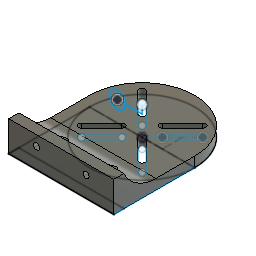
panto (Autodesk Fusion 360 archive; units mm, degrees)
design "support"
Autodesk Fusion 360 part; units mm, degrees
sketch "Esquisse1" plane through (0, 0, 0) normal (0, 1, 0) x (1, 0, 0)
  circle A0 centre (0, 0) radius 26
  line L0 (0, 0) -> (-26, 0) construction
  line L1 (0, 0) -> (26, 0) construction
  line L2 (-26, 0) -> (26, 0)
  line L3 (26, 0) -> (26, -40)
  line L4 (26, -40) -> (-26, -40)
  line L5 (-26, -40) -> (-26, 0)
  line L6 (-26, -40) -> (26, -40)
  line L7 (26, -40) -> (26, -35)
  line L8 (26, -35) -> (-26, -35)
  line L9 (-26, -35) -> (-26, -40)
  line L10 (0, 0) -> (15, 15)
  line L11 (13.9393, 16.0607) -> (3.9393, 6.0607)
  arc A1 (3.9393, 6.0607) -> (6.0607, 3.9393) centre (5, 5) ccw
  line L12 (6.0607, 3.9393) -> (16.0607, 13.9393)
  arc A2 (16.0607, 13.9393) -> (13.9393, 16.0607) centre (15, 15) ccw
  line L13 (15, 15) -> (5, 5) construction
  line L14 (0, 0) -> (10, 0) construction
  line L15 (10, 0) -> (10, 10) construction
  line L16 (-3.9393, 6.0607) -> (-13.9393, 16.0607)
  arc A3 (-6.0607, 3.9393) -> (-3.9393, 6.0607) centre (-5, 5) ccw
  line L17 (-16.0607, 13.9393) -> (-6.0607, 3.9393)
  arc A4 (-13.9393, 16.0607) -> (-16.0607, 13.9393) centre (-15, 15) ccw
  line L18 (-6.0607, -3.9393) -> (-16.0607, -13.9393)
  arc A5 (-3.9393, -6.0607) -> (-6.0607, -3.9393) centre (-5, -5) ccw
  line L19 (-13.9393, -16.0607) -> (-3.9393, -6.0607)
  arc A6 (-16.0607, -13.9393) -> (-13.9393, -16.0607) centre (-15, -15) ccw
  line L20 (3.9393, -6.0607) -> (13.9393, -16.0607)
  arc A7 (6.0607, -3.9393) -> (3.9393, -6.0607) centre (5, -5) ccw
  line L21 (16.0607, -13.9393) -> (6.0607, -3.9393)
  arc A8 (13.9393, -16.0607) -> (16.0607, -13.9393) centre (15, -15) ccw
  dimension "d1" = 52
  dimension "d2" = 40
  dimension "d3" = 5
  dimension "d4" = 3
  dimension "d5" = 10
  dimension "d7" = 360
  constraint coincident A0.centre L0.start
  constraint coincident A0 L0.end
  constraint horizontal L0
  constraint coincident A0 L1.end
  constraint parallel L0 L1
  constraint horizontal L2
  constraint vertical L3
  constraint horizontal L4
  constraint vertical L5
  constraint horizontal L6
  constraint vertical L7
  constraint horizontal L8
  constraint vertical L9
  constraint coincident L3 L7.end
  constraint tangent L11 A1
  constraint tangent A1 L12
  constraint parallel L11 L12
  constraint tangent L12 A2
  constraint tangent L11 A2
  constraint coincident L10 A1.centre
  constraint parallel L10 L13
  constraint coincident L10.end A2.centre
  constraint parallel L1 L14
  constraint midpoint L13 L15.end
  constraint perpendicular L14 L15
  measures "d1" diameter of A0
  measures "d2" distance of L0.end L4.end
  measures "d3" distance of L4.end L8.end
  measures "d4" diameter of A1
  measures "d5" distance of A0.centre L14.end
extrude "Extrusion1" add sketch "Esquisse1" along normal blind 5 contours A0 L2 | A0 L3 L5 L8 | A0 L2
extrude "Extrusion2" add sketch "Esquisse1" along normal blind 15 contours L3 L4 L5 L6 L7 L8 L9
fillet "Congé1" radius 17.5 1 edges at (0, 5, 35)
sketch "Esquisse2" plane through (0, 0, 0) normal (0, 0, 1) x (1, 0, 0)
  line L0 (0, 10) -> (-12.25, 10)
  circle A0 centre (-12.25, 10) radius 1.5
  circle A1 centre (-12.25, 10) radius 4
  line L1 (0, 10) -> (0, 14)
  dimension "d14" = 12.25
  dimension "d15" = 3
  dimension "d16" = 8
  constraint horizontal L0
  constraint coincident L0.end A0.centre
  constraint concentric A0 A1
  constraint perpendicular L0 L1
  measures "d14" distance of L0.start L0.end
  measures "d15" diameter of A0
  measures "d16" diameter of A1
extrude "Extrusion3" cut sketch "Esquisse2" along normal blind 73 contours A0
extrude "Extrusion4" cut sketch "Esquisse2" along normal blind 35
mirror "Symétrie miroir1" about plane through (0, 0, 0) normal (1, 0, 0) of "Extrusion4"
mirror "Symétrie miroir2" about plane through (0, 0, 0) normal (1, 0, 0) of "Extrusion3"
equation "d2 = 66 mm - 26 mm"

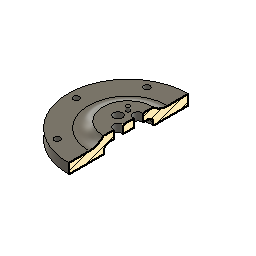
design "liaison"
Autodesk Fusion 360 part; units mm, degrees
sketch "Esquisse1" plane through (0, 0, 0) normal (0, 1, 0) x (1, 0, 0)
  circle A0 centre (5, 0) radius 2.25
  circle A1 centre (12.7279, 12.7279) radius 3
  spline S0 degree 3 poles (12.0292, -14.0552) (11.9758, -14.0271) (11.9242, -13.9959) (11.7208, -13.8551) (11.5886, -13.7213) (11.3733, -13.402) (11.2964, -13.2175) (11.2197, -12.8368) (11.2181, -12.6441) (11.2823, -12.2958) (11.3379, -12.1407) (11.4634, -11.9156) (11.5166, -11.8383) (11.5925, -11.7474) (11.6089, -11.7288) (11.6353, -11.7002) (11.645, -11.6899) (11.6633, -11.6711) (11.6718, -11.6626) (11.6907, -11.6442) (11.7011, -11.6344) (11.7308, -11.607) (11.7504, -11.5899) (11.8478, -11.5091) (11.9313, -11.453) (12.1389, -11.3418) (12.2659, -11.2945) (12.5542, -11.2293) (12.7157, -11.2194) (13.0535, -11.2528) (13.2275, -11.3022) (13.5284, -11.4499) (13.6568, -11.5398) (13.8842, -11.7592) (13.9807, -11.8877) (14.0552, -12.0292) knots 0 0 0 0 0.01809 0.01809 0.074223 0.074223 0.134132 0.134132 0.192066 0.192066 0.241514 0.241514 0.269661 0.269661 0.27709 0.27709 0.281347 0.281347 0.284952 0.284952 0.28925 0.28925 0.29707 0.29707 0.327237 0.327237 0.368009 0.368009 0.41678 0.41678 0.471117 0.471117 0.518092 0.518092 0.566073 0.566073 0.566073 0.566073
  circle A2 centre (12.7279, -12.7279) radius 3
  circle A3 centre (0, -5) radius 2.25
  arc A4 (12.0292, 14.0552) -> (-12.0292, 14.0552) centre (0, 0) ccw
  arc A5 (-14.0552, 12.0292) -> (-14.0552, -12.0292) centre (0, 0) ccw
  arc A6 (12.0292, -14.0552) -> (14.0552, -12.0292) centre (12.7279, -12.7279) ccw
  arc A7 (12.0292, -14.0552) -> (14.0552, -12.0292) centre (12.7279, -12.7279) ccw
  circle A8 centre (0, 5) radius 2.25
  arc A9 (14.0552, 12.0292) -> (12.0292, 14.0552) centre (12.7279, 12.7279) ccw
  circle A10 centre (-4.5962, 4.5962) radius 0.95
  circle A11 centre (-5, 0) radius 2.25
  arc A12 (-14.0552, -12.0292) -> (-12.0292, -14.0552) centre (-12.7279, -12.7279) ccw
  circle A13 centre (4.5962, -4.5962) radius 0.95
  circle A14 centre (0, 0) radius 12.5
  arc A15 (-12.0292, -14.0552) -> (12.0292, -14.0552) centre (0, 0) ccw
  arc A16 (14.0552, -12.0292) -> (14.0552, 12.0292) centre (0, 0) ccw
  arc A17 (-12.0292, 14.0552) -> (-14.0552, 12.0292) centre (-12.7279, 12.7279) ccw
  circle A18 centre (-12.7279, 12.7279) radius 3
  circle A19 centre (-12.7279, -12.7279) radius 3
  circle A20 centre (0, 0) radius 26
  circle A21 centre (26, 0) radius 1.5
  circle A22 centre (13, 22.5167) radius 1.5
  circle A23 centre (-13, 22.5167) radius 1.5
  circle A24 centre (-26, 0) radius 1.5
  circle A25 centre (-13, -22.5167) radius 1.5
  circle A26 centre (13, -22.5167) radius 1.5
  circle A27 centre (0, 0) radius 30
  circle A28 centre (0, 0) radius 5
  line L0 (0, 0) -> (4.5962, -4.5962)
  point P0 (-15.8247, 8.0318)
  dimension "d2" = 360
  dimension "d3" = 6
  dimension "d4" = 52
  dimension "d5" = 3
  dimension "d7" = 360
  dimension "d18" = 10
  constraint concentric A2 A7
  constraint concentric A14 A20
  constraint coincident A20 A21.centre
  constraint concentric A20 A27
  constraint concentric A14 A28
  constraint coincident A0.centre A28
  constraint coincident A11.centre A28
  constraint coincident A8.centre A28
  constraint coincident A3.centre A28
  constraint coincident A4.centre A5.centre
  constraint coincident A13.centre L0.end
  measures "d3" diameter of A2
  measures "d4" diameter of A20
  measures "d5" diameter of A21
  measures "d18" diameter of A28
extrude "Extrusion1" add sketch "Esquisse1" along normal blind 5 contours A0 A3 A8 A11 A28 | A1 A4 A9 A16 | A1 A4 A9 A16 | A1 A2 A4 A5 A15 A16 A18 A19 | A4 A5 A17 A18 | A4 A5 A17 A18 | S0 A2 A15 A16 | A2 A6 A7 A15 A16 | S0 A6 A7 | A5 A12 A15 A19 | A5 A12 A15 A19 | A14 | A20 A21 A22 A23 A24 A25 A26 | A27
extrude "Extrusion2" add sketch "Esquisse1" along normal blind 8 contours A0 A3 A8 A11 A28 | A14
fillet "Congé1" radius 10 1 edges at (-11.6541, 5, -4.5202)
extrude "Extrusion3" add sketch "Esquisse1" along normal blind 10 contours A10 | A13
extrude "Extrusion4" cut sketch "Esquisse1" along normal blind 4 contours A0 A3 A8 A11 A28 | A10 | A13 | A14
fillet "Congé2" radius 2.5 1 edges at (-11.6541, 4, 4.5202)
